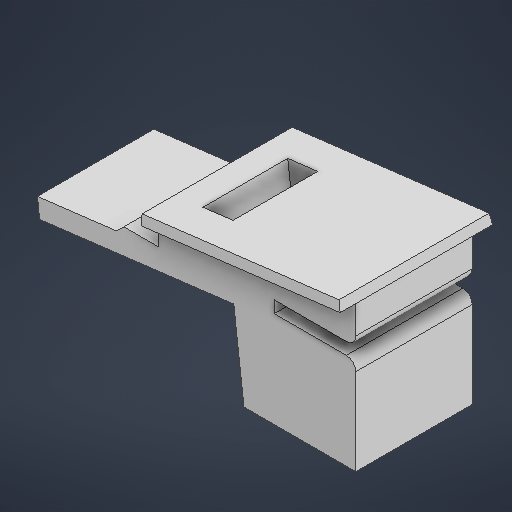
# Autodesk Inventor part: USB-C-Holder
Saved by Autodesk Inventor 2025 (Build 290162010, 162A)
## iProperties
Created: 2024-09-20
Part Number: USB-C-Holder
Material: Generic
Document SubType Name: Modeling
Designer: FizzyApple12
Density: 1 g/cm^3
Appearance: Default
Author: FizzyApple12
Autodesk Inventor part; units mm, degrees
ref_plane "YZ Plane" through (0, 0, 0) normal (1, 0, 0) x (0, 1, 0)
ref_plane "XZ Plane" through (0, 0, 0) normal (0, 1, 0) x (-1, 0, 0)
ref_plane "XY Plane" through (0, 0, 0) normal (0, 0, 1) x (1, 0, 0)
sketch "Sketch1" plane through (0, 0, 0) normal (0, 1, 0) x (-1, 0, 0)
  line L0 (0, 0) -> (-20.828, 0)
  line L1 (-20.828, 0) -> (-20.828, -12.319)
  line L2 (-20.828, -12.319) -> (0, -12.319)
  line L3 (0, -12.319) -> (0, 0)
  dimension "d0" = 20.828
  dimension "d1" = 12.319
  constraints: 8 end point, 2 parallel, 1 horizontal, 1 perpendicular
  measures "d0" distance of L2.end L1.end
  measures "d1" distance of L1.end L0.end
extrude "Extrusion1" add sketch "Sketch1" along normal blind 16.637
ref_plane "Work Plane1" through (20.828, 16.637, 0) normal (-0.1210551, 0.9926458, 0) x (0, 0, -1)
sketch "Sketch2" plane through (20.828, 16.637, 0) normal (-0.1210551, 0.9926458, 0) x (0, 0, -1)
  line L0 (14.3951, 21.2205) -> (-1.3244, 21.2205)
  line L1 (-1.3244, 21.2205) -> (-1.3244, -0.6313)
  line L2 (-1.3244, -0.6313) -> (14.3951, -0.6313)
  line L3 (14.3951, -0.6313) -> (14.3951, 21.2205)
  point P0 (0, 22.6888)
  constraints: 8 end point, 2 parallel, 1 horizontal, 1 perpendicular
extrude "Extrusion2" cut sketch "Sketch2" along normal blind 16.637
sketch "Sketch3" plane through (20.828, 16.637, 0) normal (-0.1210551, 0.9926458, 0) x (0.9926458, 0.1210551, 0)
  line L0 (0, 0) -> (-20.9823, 0) projected
  line L1 (0, 0) -> (0, 12.319) projected
  line L2 (-20.9823, 12.319) -> (0, 12.319) projected
  line L3 (-20.9823, 0) -> (-20.9823, 12.319) projected
  line L4 (-20.9823, 14.097) -> (0, 14.097)
  line L5 (0, 14.097) -> (0, -1.778)
  line L6 (0, -1.778) -> (-20.9823, -1.778)
  line L7 (-20.9823, -1.778) -> (-20.9823, 14.097)
  line L8 (-20.9823, 0) -> (-20.9823, 12.319) projected
  point P0 (-22.6888, 0)
  point P1 (-20.9823, 6.1595)
  dimension "d9" = 15.875
  constraints: 8 end point, 2 collinear, 2 midpoint, 2 parallel, 1 horizontal, 1 perpendicular
  measures "d9" distance between parallel lines of L6 L4
extrude "Extrusion3" add sketch "Sketch3" against normal blind 1.016 draft 6.953
ref_plane "Work Plane2" through (0, 11.43, 0) normal (0, -1, 0) x (1, 0, 0)
sketch "Sketch4" plane through (0, 11.43, 0) normal (0, -1, 0) x (1, 0, 0)
  line L0 (20.828, 0) -> (20.828, -12.319) projected
  line L1 (0, 0) -> (20.828, 0) projected
  line L2 (0, -12.319) -> (0, 0) projected
  line L3 (20.828, -12.319) -> (0, -12.319) projected
  line L4 (20.828, 0) -> (12.192, 0)
  line L5 (12.192, 0) -> (12.192, -12.319)
  line L6 (12.192, -12.319) -> (20.828, -12.319)
  line L7 (20.828, -12.319) -> (20.828, 0)
  point P0 (20.828, -6.1595)
  dimension "d11" = 8.636
  constraints: 8 end point, 2 midpoint, 2 parallel, 1 collinear, 1 horizontal, 1 perpendicular
  measures "d11" distance between parallel lines of L7 L5
extrude "Extrusion4" cut sketch "Sketch4" along normal blind 1.27 contours L0 L3 L5 L1
sketch "Sketch5" plane through (0, 11.43, 0) normal (0, -1, 0) x (1, 0, 0)
  line L0 (0, -12.319) -> (0, 0) projected
  line L1 (-5.715, 0) -> (0, 0)
  line L2 (0, 0) -> (0, -12.319)
  line L3 (0, -12.319) -> (-5.715, -12.319)
  line L4 (-5.715, -12.319) -> (-5.715, 0)
  dimension "d14" = 5.715
  constraints: 8 end point, 2 parallel, 1 horizontal, 1 perpendicular
  measures "d14" distance between parallel lines of L0 L4
extrude "Extrusion5" add sketch "Sketch5" along normal up to surface (11.43 mm away)
extrude "Extrusion6" cut sketch "Sketch5" along normal blind 1.27
chamfer "Chamfer1" distance 2 angle 45 1 edges at (-5.715, 10.16, -6.1595)
fillet "Fillet1" radius 1 2 edges at (20.828, 10.16, -6.1595) (20.828, 11.43, -6.1595)
sketch "Sketch6" plane through (20.828, 16.637, 0) normal (-0.1210551, 0.9926458, 0) x (0.9926458, 0.1210551, 0)
  line L0 (-17.9823, 10.6426) -> (-14.7819, 10.6426)
  line L1 (-14.7819, 10.6426) -> (-14.7819, 1.6764)
  line L2 (-14.7819, 1.6764) -> (-17.9823, 1.6764)
  line L3 (-17.9823, 1.6764) -> (-17.9823, 10.6426)
  line L4 (-17.9823, 6.1595) -> (-20.9823, 6.1595) construction
  line L5 (-20.9823, 14.097) -> (-20.9823, -1.778) construction
  point P0 (-22.6888, 0)
  dimension "d23" = 3.2004
  dimension "d24" = 8.9662
  dimension "d25" = 3
  constraints: 10 end point, 2 midpoint, 2 parallel, 2 perpendicular, 1 horizontal
  measures "d23" distance of L1.end L2.end
  measures "d24" distance of L0.end L1.end
  measures "d25" distance of L4.start L4.end
extrude "Extrusion7" cut sketch "Sketch6" against normal blind 6.1214
sketch "Sketch7" plane through (21.569, 10.5606, 0) normal (-0.1210551, 0.9926458, 0) x (0.9926458, 0.1210551, 0)
  line L0 (-39.5219, 14.9352) -> (-14.7569, 14.9352)
  line L1 (-14.7569, 14.9352) -> (-14.7569, -0.8636)
  line L2 (-14.7569, -0.8636) -> (-39.5219, -0.8636)
  line L3 (-39.5219, -0.8636) -> (-39.5219, 14.9352)
  line L4 (-39.5219, 14.9352) -> (-14.7569, 14.9352)
  line L5 (-14.7569, 14.9352) -> (-14.7569, 18.1864)
  line L6 (-14.7569, 18.1864) -> (-39.5219, 18.1864)
  line L7 (-39.5219, 18.1864) -> (-39.5219, 14.9352)
  line L8 (-14.7819, 10.6426) -> (-14.7819, 1.6764) construction
  line L9 (-14.7819, 1.6764) -> (-17.9823, 1.6764) construction
  line L10 (-2.014, 0) -> (-2.014, 12.319) construction
  line L11 (-2.014, 0) -> (-28.3618, 0) construction
  line L12 (-28.3618, 0) -> (-28.3618, 12.319) construction
  line L13 (-2.014, 12.319) -> (-28.3618, 12.319) construction
  line L14 (-14.7569, 0) -> (-34.4419, 0)
  line L15 (-34.4419, 0) -> (-34.4419, 12.319)
  line L16 (-34.4419, 12.319) -> (-14.7569, 12.319)
  line L17 (-14.7569, 12.319) -> (-14.7569, 0) construction
  line L18 (-14.7819, 1.6764) -> (-17.9823, 1.6764) projected
  line L19 (-14.7819, 10.6426) -> (-14.7819, 1.6764) projected
  line L20 (-17.9823, 10.6426) -> (-14.7819, 10.6426) projected
  line L21 (-17.9823, 1.6764) -> (-17.9823, 10.6426) projected
  line L22 (-14.7569, 18.1864) -> (-13.7569, 18.1864)
  line L23 (-13.7569, 18.1864) -> (-13.7569, -0.8636)
  line L24 (-13.7569, -0.8636) -> (-14.7569, -0.8636)
  line L25 (-14.7569, -0.8636) -> (-14.7569, 18.1864)
  point P0 (-22.6888, 0)
  point P1 (-14.7569, 12.319)
  dimension "d28" = 24.765
  dimension "d29" = 15.7988
  dimension "d30" = 19.05
  dimension "d31" = 0.025
  dimension "d32" = 2.54
  dimension "d35" = 5.08
  dimension "d38" = 1
  constraints: 32 end point, 8 parallel, 4 horizontal, 4 perpendicular, 3 point on line
  measures "d28" distance of L1.end L2.end
  measures "d29" distance of L1.end L0.end
  measures "d30" distance between parallel lines of L6 L2
  measures "d31" distance between parallel lines of L8 L1
  measures "d32" distance between parallel lines of L9 L2
  measures "d35" distance between parallel lines of L15 L3
  measures "d38" distance between parallel lines of L5 L23
extrude "Extrusion8" cut sketch "Sketch7" against normal through all contours L7 L6 L5 L0 | L0 L1 L16 L15 L14 L2 L3 | L5 L22 L23 L24 L1 | L1 L14 L15 L16 | L18 L21 L20 L19
extrude "Extrusion9" add sketch "Sketch7" along normal blind 2 contours L1 L14 L15 L16
chamfer "Chamfer2" distance 1 angle 45 1 edges at (3.719, 8.3838, -6.1595)
body "Solid1"
